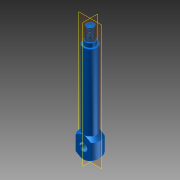
# Autodesk Inventor part: TU-006
Saved by Autodesk Inventor 2011 (Build 150229000, 229)
## iProperties
Shininess: 64.0
Angle Display Precision: 2
Document Length Units: 11269
Document Angle Units: 11279
Document Time Units: 11290
Document Mass Units: 11286
Document Length Units Precision: 3
Document Angle Units Precision: 2
Compacted: True
Created: 2002-07-24
Part Number: TU-006
Document SubType Name: Modeling
Designer: PN
Description: Piston Rod
Density: 8.08 g/cm^3
Mass: 144.065 g
Surface Area: 58.412 cm^2
Volume: 17.8299 cm^3
Material: Stainless Steel
Density: 0.0
Volumn: 0.0
Area: 0.0
PropertySet Name: Model Information
Control State: 0
Master: False
Checked Out: False
LENGTH: 1.000 in
Author: PN
Autodesk Inventor part; units mm, degrees
ref_plane "XZ Plane" through (0, 0, 0) normal (0, 1, 0) x (-1, 0, 0)
sketch "Sketch1" plane through (0, 0, 0) normal (0, 0, 1) x (1, 0, 0)
  line L0 (10.5, 0) -> (0, 0)
  line L1 (0, 117) -> (4, 117)
  line L2 (4, 117) -> (4, 104)
  line L3 (4, 104) -> (5, 104)
  line L4 (5, 104) -> (5, 100)
  line L5 (5, 100) -> (7, 100)
  line L6 (7, 100) -> (7, 22)
  line L7 (10.5, 22) -> (10.5, 0)
  line L8 (0, 117) -> (0, 0)
  line L9 (7, 22) -> (10.5, 22)
  dimension "d10" = 21
  dimension "d11" = 14
  dimension "d12" = 22
  dimension "d13" = 100
  dimension "d14" = 104
  dimension "d15" = 117
  dimension "d16" = 8
  dimension "d17" = 10
  constraints: 20 end point, 6 parallel, 3 perpendicular, 1 coincident, 1 vertical
  measures "d10" diameter of L7 L8
  measures "d11" diameter of L6 L8
  measures "d12" distance of L7.start L0.start
  measures "d13" distance from line of L6.start L0
  measures "d14" distance between parallel lines of L3 L0
  measures "d15" distance between parallel lines of L0 L1
  measures "d16" diameter of L2 L8
  measures "d17" diameter of L4 L8
revolve "Revolution1" add sketch "Sketch1" angle 360 about axis through (0, 117, 0) along (0, -1, 0)
sketch "Sketch2" plane through (0, 0, 0) normal (0, 0, 1) x (1, 0, 0)
  line L0 (-10.5, 22) -> (-10.5, 0) projected
  line L1 (10.5, 22) -> (10.5, 0) projected
  line L2 (-10.5, 11) -> (10.5, 11) construction
  circle A0 centre (0, 11) radius 4 construction
  dimension "d1" = 8
  constraints: 3 midpoint, 2 end point, 1 centre point
  measures "d1" diameter of A0
ref_plane "Work Plane1" through (0, 11, 10.5) normal (0, 0, 1) x (1, 0, 0)
sketch "Sketch3" plane through (0, 11, 10.5) normal (0, 0, 1) x (1, 0, 0)
  point P0 (0, -11)
  point P1 (0, 0)
hole "Hole1" at (0, 11, 10.5) direction (0, 0, -1) diameter 8 end through all
ref_plane "Work Plane2" through (0, 61, 7) normal (0, 0, 1) x (1, 0, 0)
sketch "Sketch4" plane through (0, 61, 7) normal (0, 0, 1) x (1, 0, 0)
  line L0 (-10.5, -39) -> (10.5, -39) projected
  line L1 (-10.5, -61) -> (10.5, -61) projected
  line L2 (-10.5, -61) -> (-10.5, -39)
  line L3 (10.5, -61) -> (10.5, -39)
  point P0 (0, -61)
  constraints: 4 end point, 1 parallel, 1 perpendicular
extrude "Extrusion1" cut sketch "Sketch4" along normal through all
mirror "Mirror1" about plane through (0, 0, 0) normal (0, 0, 1) of "Extrusion1"
chamfer "Chamfer1" distance 3.5 angle 45 4 edges at (10.5, 22, 0) (-10.5, 22, 0) (10.5, 0, 0) (-10.5, 0, 0)
thread "Thread1" size "M8x1" class "6g" standard "ANSI Metric M Profile" full length
equation "\"LENGTH\" = 25.4"
body "Solid1"
